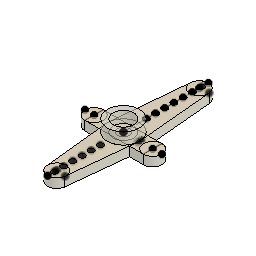
OttoDIY_v09 (Autodesk Fusion 360 archive; units mm, degrees)
design "Servo_SG90_cross"
Autodesk Fusion 360 part; units mm, degrees
sketch "Sketch1" plane through (0, 0, 0) normal (0, 0, 1) x (1, 0, 0)
  circle A0 centre (0, 0) radius 3.5
  circle A1 centre (0, 0) radius 2.25
  circle A2 centre (0, 16.5) radius 2
  circle A3 centre (0, -14.5) radius 2
  circle A4 centre (-6.375, 0) radius 2
  circle A5 centre (6.375, 0) radius 2
  line L0 (0, 0) -> (0, 16.5) construction
  line L1 (-1.9917, 16.6818) -> (-3.4855, 0.3182)
  line L2 (-1.9893, -14.7069) -> (-3.4812, -0.3621)
  line L3 (1.9917, 16.6818) -> (3.4855, 0.3182)
  line L4 (1.9893, -14.7069) -> (3.4812, -0.3621)
  line L5 (-6.375, 2) -> (6.375, 2)
  line L6 (6.375, 2) -> (6.375, -2) construction
  line L7 (6.375, -2) -> (-6.375, -2)
  line L8 (-6.375, -2) -> (-6.375, 2) construction
  circle A6 centre (0, 0) radius 1.25
  circle A7 centre (0, 5) radius 0.625
  circle A8 centre (0, 7) radius 0.625
  circle A9 centre (0, 9) radius 0.625
  circle A10 centre (0, 11) radius 0.625
  circle A11 centre (0, 13) radius 0.625
  circle A12 centre (0, 15) radius 0.625
  circle A13 centre (0, 17) radius 0.625
  circle A14 centre (0, -5) radius 0.625
  circle A15 centre (0, -7) radius 0.625
  circle A16 centre (0, -9) radius 0.625
  circle A17 centre (0, -11) radius 0.625
  circle A18 centre (0, -13) radius 0.625
  circle A19 centre (0, -15) radius 0.625
  point P0 (0, -16.5)
  point P1 (0, 18.5)
  point P2 (-8.375, 0)
  point P3 (8.375, 0)
  dimension "d1" = 7
  dimension "d2" = 4.5
  dimension "d5" = 35
  dimension "d7" = 4
  dimension "d8" = 16.75
  dimension "d9" = 14.5
  dimension "d12" = 2.5
  dimension "d14" = 5
  dimension "d15" = 1.25
  dimension "d16" = 2
  dimension "d17" = 2
  dimension "d18" = 2
  dimension "d19" = 2
  dimension "d20" = 2
  dimension "d21" = 2
  dimension "d22" = 5
  dimension "d23" = 2
  dimension "d24" = 2
  dimension "d25" = 2
  dimension "d26" = 2
  dimension "d27" = 2
  constraint coincident A0.centre A1.centre
  constraint vertical A0.centre A3.centre
  constraint vertical A0.centre A2.centre
  constraint coincident A3 P0
  constraint coincident A2 P1
  constraint vertical A3.centre P0
  constraint equal A2 A3
  constraint equal A3 A4
  constraint equal A3 A5
  constraint horizontal A0.centre A5.centre
  constraint coincident A4 P2
  constraint coincident A5 P3
  constraint horizontal A4.centre P2
  constraint horizontal A5.centre P3
  constraint coincident A2.centre L0.end
  constraint symmetric P2 P3 L0
  constraint coincident A2 L1.start
  constraint coincident A0 L1.end
  constraint tangent A2 L1
  constraint tangent A0 L1
  constraint coincident A3 L2.start
  constraint coincident A0 L2.end
  constraint tangent A3 L2
  constraint tangent A0 L2
  constraint symmetric L0 L1.start L3.start
  constraint symmetric L0 L1.end L3.end
  constraint symmetric L0 L2.start L4.start
  constraint symmetric L0 L2.end L4.end
  constraint horizontal L5
  constraint vertical L6
  constraint horizontal L7
  constraint vertical L8
  constraint coincident A5 L6.end
  constraint coincident A4 L5.start
  constraint coincident A5.centre L6
  constraint coincident A4.centre L8
  constraint coincident L0 A7.centre
  constraint coincident L0 A8.centre
  constraint coincident L0 A9.centre
  constraint coincident L0 A10.centre
  constraint coincident L0 A11.centre
  constraint coincident L0 A12.centre
  constraint equal A7 A8
  constraint equal A7 A9
  constraint equal A7 A10
  constraint equal A7 A11
  constraint equal A7 A12
  constraint equal A7 A13
  constraint vertical A2.centre A13.centre
  constraint equal A7 A14
  constraint equal A7 A15
  constraint equal A7 A16
  constraint equal A7 A17
  constraint equal A7 A18
  constraint equal A7 A19
  constraint vertical A18.centre A19.centre
  constraint vertical A17.centre A18.centre
  constraint vertical A15.centre A16.centre
  constraint vertical A16.centre A17.centre
  constraint vertical A14.centre A15.centre
  constraint vertical A0.centre A14.centre
  measures "d1" diameter of A0
  measures "d2" diameter of A1
  measures "d5" distance of P0 P1
  measures "d7" diameter of A3
  measures "d8" horizontal distance of P2 P3
  measures "d9" distance of A0.centre A3.centre
  measures "d12" diameter of A6
  measures "d14" distance of A0.centre A7.centre
  measures "d15" diameter of A7
  measures "d16" distance of A7.centre A8.centre
  measures "d17" distance of A8.centre A9.centre
  measures "d18" distance of A9.centre A10.centre
  measures "d19" distance of A10.centre A11.centre
  measures "d20" distance of A11.centre A12.centre
  measures "d21" vertical distance of A12.centre A13.centre
  measures "d22" distance of A0.centre A14.centre
  measures "d23" distance of A14.centre A15.centre
  measures "d24" distance of A15.centre A16.centre
  measures "d25" distance of A16.centre A17.centre
  measures "d26" distance of A17.centre A18.centre
  measures "d27" distance of A18.centre A19.centre
extrude "Extrude1" add sketch "Sketch1" along normal blind 2.5 contours A0 A1 L5 L7 | A0 A1 L5 | A0 A1 L7 | A0 A1 L5 L7
extrude "Extrude2" add sketch "Sketch1" against normal blind 2 contours A0 A1 L5 L7 | A0 A5 L3 L4 L5 L7 | A0 L3 L5 | A0 L4 L7 | A0 A1 L5 | A0 A2 L1 L3 L5 A12 | A0 A3 L2 L4 L7 A18 | A0 A1 L7 | A0 A1 L5 L7 | A0 L1 L5 | A1 L5 | A1 L5 L7 | A2 A12 | A5 | A0 L2 L7 | A1 L7 | A3 A18 | A0 A4 L1 L2 L5 L7 | A4 | A2 A12 | A2 A12 | A3 A18 | A3 A18 | A6 | A7 | A8 | A9 | A10 | A11 | A13 | A14 | A15 | A16 | A17 | A19
extrude "Extrude3" cut sketch "Sketch1" against normal through all contours A2 A12 | A2 A12 | A3 A18 | A3 A18 | A6 | A7 | A8 | A9 | A10 | A11 | A13 | A14 | A15 | A16 | A17 | A19 picked at (-0.0144, 14.4623) picked at (-0.0082, 14.8783) picked at (0.0144, -12.4623) picked at (-0.0082, -12.8783)
